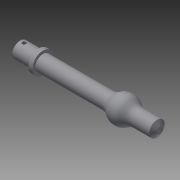
# Autodesk Inventor part: Shifting Shaft
Saved by Autodesk Inventor 2013 (Build 170138000, 138)
## iProperties
Created: 2013-06-06
Part Number: Shifting Shaft
Material: Generic
Document SubType Name: Modeling
Designer: mvarma
Density: 1 g/cm^3
Author: mvarma
Autodesk Inventor part; units mm, degrees
ref_plane "YZ Plane" through (0, 0, 0) normal (1, 0, 0) x (0, 1, 0)
ref_plane "XZ Plane" through (0, 0, 0) normal (0, 1, 0) x (-1, 0, 0)
ref_plane "XY Plane" through (0, 0, 0) normal (0, 0, 1) x (1, 0, 0)
sketch "Sketch1" plane through (0, 0, 0) normal (0, 0, 1) x (1, 0, 0)
  line L0 (0, 0) -> (0, 3.1115)
  line L1 (0, 5.5562) -> (26.1938, 5.5563) construction
  line L2 (0, 7.9375) -> (26.1938, 7.9375) construction
  line L3 (26.1938, 7.9375) -> (26.1938, 5.5563) construction
  line L4 (26.1938, 5.5563) -> (26.1938, 0) construction
  line L5 (26.1938, 0) -> (24.6063, 0) construction
  line L6 (26.1938, 6.35) -> (34.3853, 6.35) construction
  line L7 (26.1938, 0) -> (34.3853, 0) construction
  line L8 (34.3853, 0) -> (34.3853, 6.35) construction
  line L9 (16.6688, 7.9375) -> (16.6688, 0) construction
  circle A0 centre (16.6688, 7.5565) radius 2.3813 construction
  circle A1 centre (16.6688, 5.4928) radius 2.3813 construction
  circle A2 centre (10.3188, 7.5565) radius 2.3813 construction
  circle A3 centre (10.3188, 5.4928) radius 2.3813 construction
  line L10 (10.3188, 7.9375) -> (10.3188, 0) construction
  line L11 (0, 5.1753) -> (8.7313, 5.1753) construction
  line L12 (8.7313, 5.1753) -> (8.7313, 0) construction
  line L13 (5.5563, 5.1753) -> (5.5563, 0) construction
  line L14 (18.2563, 5.1753) -> (18.2563, 0) construction
  line L15 (21.4313, 5.1753) -> (21.4313, 0) construction
  line L16 (0, 3.1115) -> (5.5563, 3.1115)
  line L17 (5.5563, 3.1115) -> (8.7313, 5.1753)
  line L18 (18.2563, 5.1753) -> (21.4313, 3.1115) construction
  line L19 (11.9063, 5.1753) -> (11.9063, 0) construction
  line L20 (15.0813, 5.1753) -> (15.0813, 0) construction
  line L21 (11.9063, 5.1753) -> (15.0813, 3.1115)
  line L22 (21.4313, 3.3734) -> (34.3853, 3.3734) construction
  line L23 (24.6063, 3.3734) -> (24.6063, 1.321) construction
  line L24 (21.4313, 3.3734) -> (20.1197, 5.5563) construction
  line L25 (26.1938, 3.1115) -> (30.9563, 3.1115) construction
  line L26 (30.9563, 3.1115) -> (30.9563, 0) construction
  line L27 (31.75, 3.3734) -> (31.75, 0) construction
  line L28 (31.75, 0) -> (29.723, 3.3734) construction
  line L29 (0, 7.9375) -> (-1.5875, 7.9375) construction
  line L30 (-1.5875, 7.9375) -> (-1.5875, 3.3734) construction
  line L31 (-1.5875, 3.3734) -> (5.5563, 3.3734) construction
  line L32 (5.5563, 3.1115) -> (15.0813, 3.1115) construction
  line L33 (15.0813, 3.1115) -> (23.5304, 3.1115)
  line L34 (11.9063, 5.1753) -> (26.1938, 5.1753) construction
  line L35 (8.7313, 5.1753) -> (11.9063, 5.1753)
  line L36 (24.6063, 3.1115) -> (26.1938, 3.1115) construction
  line L37 (24.6063, 1.321) -> (23.5304, 3.1115)
  line L38 (25.4, 0) -> (25.4, 3.3734) construction
  line L39 (24.6063, 1.321) -> (24.6063, 0)
  line L40 (23.5304, 3.1115) -> (24.6063, 3.1115) construction
  line L41 (0, 3.1115) -> (0, 12.7) construction
  line L42 (24.6063, 0) -> (0, 0)
  line L43 (24.6063, 1.321) -> (25.4, 0) construction
  point P0 (0, 0)
  dimension "d0" = 12.7
  dimension "d1" = 5.5563
  dimension "d2" = 7.9375
  dimension "d3" = 26.1938
  dimension "d4" = 8.1915
  dimension "d5" = 6.35
  dimension "d6" = 9.525
  dimension "d7" = 6.35
  dimension "d8" = 0.381
  dimension "d9" = 0.381
  dimension "d10" = 0.0635
  dimension "d11" = 0.0635
  dimension "d12" = 1.5875
  dimension "d13" = 4.7625
  dimension "d14" = 1.5875
  dimension "d15" = 4.7625
  dimension "d17" = 1.5875
  dimension "d18" = 4.7625
  dimension "d19" = 3.3734
  dimension "d20" = 3.175
  dimension "d21" = 31
  dimension "d23" = 9.525
  dimension "d24" = 0.7937
  dimension "d25" = 31
  dimension "d26" = 1.5875
  dimension "d33" = 4.7625
  dimension "d35" = 31
  dimension "d36" = 3.3734
  dimension "d37" = 3.1115
  dimension "d38" = 0.7937
  dimension "d43" = 10.3187
  constraints: 84 end point, 40 point on line, 20 perpendicular, 17 vertical, 6 tangent, 4 centre point, 3 equal radius, 2 coincident, 2 collinear, 2 horizontal, 2 parallel, 23 other
  measures "d0" distance of L0.start L41.end
  measures "d1" distance from line of L1 L0.start
  measures "d2" distance from line of L0.start L2
  measures "d3" distance of L2.start L2.end
  measures "d4" distance of L6.start L6.end
  measures "d5" distance of L7.end L6.end
  measures "d6" distance between parallel lines of L3 L9
  measures "d7" distance between parallel lines of L9 L10
  measures "d8" distance from line of L2 A2.centre
  measures "d9" distance from line of L2 A0.centre
  measures "d10" distance from line of L1 A1.centre
  measures "d11" distance from line of L1 A3.centre
  measures "d12" distance between parallel lines of L12 L10
  measures "d13" distance between parallel lines of L13 L10
  measures "d14" distance between parallel lines of L9 L14
  measures "d15" distance between parallel lines of L15 L9
  measures "d17" distance between parallel lines of L10 L19
  measures "d18" distance between parallel lines of L10 L20
  measures "d19" distance between parallel lines of L7 L22
  measures "d20" distance between parallel lines of L15 L23
  measures "d21" angle of L15 L24
  measures "d23" distance from line of L26 L18.end
  measures "d24" distance between parallel lines of L27 L26
  measures "d25" angle of L27 L28
  measures "d26" distance of L2.start L29.end
  measures "d33" diameter of A2
  measures "d35" angle of L38 L37
  measures "d36" distance of the line from the sketch origin of L31
  measures "d37" distance of the line from the sketch origin of L16
  measures "d38" distance between parallel lines of L38 L23
  measures "d43" distance between parallel lines of L0 L10
revolve "Revolution1" add sketch "Sketch1" angle 360 about axis through (24.6063, 0, 0) along (-1, 0, 0)
ref_plane "Work Plane1" through (10.3188, 0, 0) normal (-1, 0, 0) x (0, 0, 1)
fillet "Fillet1" radius 3.9688 4 edges at (5.5563, -3.1115, 0) (15.0813, -3.1115, 0) (11.9063, -5.1753, 0) (8.7313, -5.1753, 0)
sketch "Sketch2" plane through (0, 0, 0) normal (-1, 0, 0) x (0, 0, 1)
  circle A0 centre (0, 0) radius 3.1115 projected
extrude "Extrusion1" add sketch "Sketch2" along normal blind 23.5394
sketch "Sketch3" plane through (0, 0, 0) normal (0, 0, 1) x (1, 0, 0)
  line L0 (-23.5394, 3.1115) -> (4.3798, 3.1115) projected
  arc A0 (4.3798, 3.1115) -> (6.5427, 3.7527) centre (4.3798, 7.0802) ccw projected
  line L1 (6.5427, 3.7527) -> (7.7448, 4.5341) projected
  arc A1 (9.9077, 5.1753) -> (7.7448, 4.5341) centre (9.9077, 1.2065) ccw projected
  line L2 (9.9077, 5.1753) -> (10.7298, 5.1753) projected
  arc A2 (12.8927, 4.5341) -> (10.7298, 5.1753) centre (10.7298, 1.2065) ccw projected
  line L3 (12.8927, 4.5341) -> (14.0948, 3.7527) projected
  arc A3 (14.0948, 3.7527) -> (16.2577, 3.1115) centre (16.2577, 7.0803) ccw projected
  line L4 (16.2577, 3.1115) -> (23.5304, 3.1115) projected
  circle A4 centre (7.5381, 9.9656) radius 2.3812
  line L5 (4.3798, 7.0802) -> (4.3798, 3.1115) construction
  line L6 (4.3798, 7.0802) -> (6.5427, 3.7527) construction
  line L7 (9.9077, 1.2065) -> (7.7448, 4.5341) construction
  line L8 (9.9077, 1.2065) -> (9.9077, 5.1753) construction
  line L9 (10.7298, 1.2065) -> (10.7298, 5.1753) construction
  line L10 (10.7298, 1.2065) -> (12.8927, 4.5341) construction
  line L11 (16.2577, 7.0803) -> (14.0948, 3.7527) construction
  line L12 (16.2577, 7.0803) -> (16.2577, 3.1115) construction
  line L13 (-5.9448, 5.4927) -> (4.3798, 5.4927)
  arc A5 (4.3798, 5.4927) -> (5.2449, 5.7492) centre (4.3798, 7.0802) ccw
  line L14 (7.7448, 4.5341) -> (6.4471, 6.5306) construction
  line L15 (5.2449, 5.7492) -> (6.4471, 6.5306)
  line L16 (9.9077, 5.1753) -> (9.9077, 7.5565) construction
  arc A6 (9.9077, 7.5565) -> (6.4471, 6.5306) centre (9.9077, 1.2065) ccw
  point P0 (0, 0)
  dimension "d45" = 4.7625
  dimension "d47" = 2.3813
  dimension "d49" = 2.3876
  constraints: 25 end point, 6 perpendicular, 4 point on circle, 3 centre point, 3 parallel, 2 coincident, 1 collinear, 1 horizontal, 1 point on line, 1 tangent
  measures "d45" diameter of A4
  measures "d47" distance between parallel lines of L0 L13
sketch "Sketch4" plane through (-23.5394, 0, 0) normal (-1, 0, 0) x (0, 0, 1)
  circle A0 centre (0, 0) radius 3.1115 projected
  circle A1 centre (0, 0) radius 4.2545
  dimension "d50" = 8.509
  constraints: 1 centre point, 1 coincident
  measures "d50" diameter of A1
extrude "Extrusion2" add sketch "Sketch4" against normal blind 1.5875
sketch "Sketch5" plane through (-23.5394, 0, 0) normal (-1, 0, 0) x (0, 0, 1)
  circle A0 centre (0, 0) radius 4.2545 projected
  circle A1 centre (0, 0) radius 3.175
  dimension "d54" = 6.35
  constraints: 1 centre point, 1 coincident
  measures "d54" diameter of A1
extrude "Extrusion3" add sketch "Sketch5" along normal blind 4.9784 contours A1
sketch "Sketch6" plane through (0, 0, 0) normal (0, 1, 0) x (-1, 0, 0)
  line L0 (28.5178, -3.175) -> (28.5178, 3.175) projected
  line L1 (23.5394, 3.175) -> (23.5394, -3.175) projected
  line L2 (23.5394, 3.175) -> (28.5178, 3.175) projected
  line L3 (23.5394, -3.175) -> (28.5178, -3.175) projected
  circle A0 centre (29.4322, 0) radius 0.7874
  line L4 (28.6448, 3.175) -> (28.6448, -3.175) construction
  line L5 (28.5178, 0) -> (29.4322, 0) construction
  line L6 (28.5178, 3.175) -> (28.6448, 3.175) construction
  line L7 (28.6448, -3.175) -> (28.5178, -3.175) construction
  line L8 (28.5178, 3.175) -> (31.0578, 3.175)
  line L9 (31.0578, 3.175) -> (31.0578, 0)
  line L10 (31.0578, -3.175) -> (28.5178, -3.175) construction
  line L11 (28.5178, 0) -> (31.0578, 0)
  line L12 (31.0578, 0) -> (31.0578, -3.175) construction
  line L13 (28.5178, 0) -> (28.5178, 3.175)
  point P0 (0, 0)
  point P1 (30.2196, 0)
  point P2 (28.6448, 0)
  dimension "d57" = 1.5748
  dimension "d58" = 0.127
  dimension "d60" = 2.54
  constraints: 20 end point, 9 perpendicular, 2 midpoint, 2 point on line, 1 coincident, 1 collinear, 1 horizontal alignment, 1 parallel, 1 vertical, 2 other
  measures "d58" distance between parallel lines of L0 L4
  measures "d60" distance between parallel lines of L12 L0
sketch "Sketch7" plane through (-28.5178, 0, 0) normal (-1, 0, 0) x (0, 0, 1)
  circle A0 centre (0, 0) radius 3.175 projected
extrude "Extrusion4" add sketch "Sketch7" along normal blind 2.54
extrude "Extrusion5" cut sketch "Sketch6" along normal through all both and the other way through all contours L11 A0 | A0 L11
equation "\"d1\" = d28"
equation "\"d2\" = d29"
equation "\"d8\" = d30"
equation "\"d9\" = d8"
equation "\"d10\" = d31"
equation "\"d11\" = d10"
equation "\"d17\" = d12"
equation "\"d18\" = d13"
equation "\"d23\" = d22"
equation "\"d25\" = d21"
equation "\"d35\" = d25"
equation "\"d44\" = -d43"
equation "\"d28\" = 5.55625"
equation "\"d29\" = 7.9375"
equation "\"d30\" = 0.381"
equation "\"d31\" = 0.0635"
equation "\"d22\" = 9.525"
body "Solid1"
